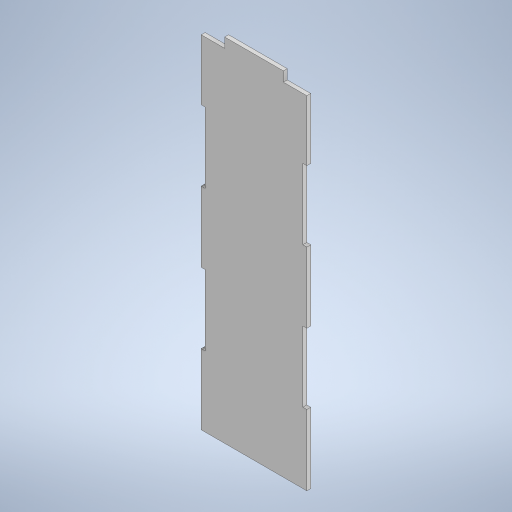
# Autodesk Inventor part: front_side
Saved by Autodesk Inventor 2023 (Build 270158000, 158)
## iProperties
Created: 2023-04-26
Part Number: front_side
Material: Generic
Document SubType Name: Modeling
Designer: Unnar
Density: 1 g/cm^3
Appearance: Default
Author: Unnar
Autodesk Inventor part; units mm, degrees
ref_plane "YZ Plane" through (0, 0, 0) normal (1, 0, 0) x (0, 1, 0)
ref_plane "XZ Plane" through (0, 0, 0) normal (0, 1, 0) x (-1, 0, 0)
ref_plane "XY Plane" through (0, 0, 0) normal (0, 0, 1) x (1, 0, 0)
sketch "Sketch1" plane through (0, 0, 0) normal (0, 0, 1) x (1, 0, 0)
  line L0 (-28.8571, 66) -> (25.1429, 66)
  line L1 (25.1429, 66) -> (25.1429, -114)
  line L2 (25.1429, -114) -> (-28.8571, -114)
  line L3 (-28.8571, -114) -> (-28.8571, 66)
  point P0 (0, 0)
  dimension "d0" = 54
  dimension "d1" = 180
  constraints: 8 end point, 2 parallel, 1 horizontal, 1 perpendicular
  measures "d0" distance of L0.start L0.end
  measures "d1" distance of L0.end L1.end
extrude "Extrusion1" add sketch "Sketch1" along normal blind 2
sketch "Sketch2" plane through (0, 0, 2) normal (0, 0, 1) x (1, 0, 0)
  line L0 (25.1429, 66) -> (-28.8571, 66) projected
  line L1 (-28.8571, 66) -> (-16.8571, 66)
  line L2 (-16.8571, 66) -> (-16.8571, 61)
  line L3 (-16.8571, 61) -> (-28.8571, 61)
  line L4 (-28.8571, 61) -> (-28.8571, 66)
  line L5 (25.1429, 66) -> (13.1429, 66)
  line L6 (13.1429, 66) -> (13.1429, 61)
  line L7 (13.1429, 61) -> (25.1429, 61)
  line L8 (25.1429, 61) -> (25.1429, 66)
  point P0 (0, 0)
  dimension "d4" = 12
  dimension "d5" = 12
  dimension "d6" = 5
  constraints: 16 end point, 4 parallel, 2 horizontal, 2 perpendicular, 1 point on line
  measures "d4" distance of L6.end L7.end
  measures "d5" distance of L2.end L3.end
  measures "d6" distance of L3.end L0.end
extrude "Extrusion2" cut sketch "Sketch2" against normal blind 2
sketch "Sketch3" plane through (0, 0, 2) normal (0, 0, 1) x (1, 0, 0)
  line L0 (-28.8571, 61) -> (-28.8571, -114) projected
  line L1 (-28.8571, 30) -> (-26.8571, 30)
  line L2 (-26.8571, 30) -> (-26.8571, -6)
  line L3 (-26.8571, -6) -> (-28.8571, -6)
  line L4 (-28.8571, -6) -> (-28.8571, 30)
  line L5 (-28.8571, -42) -> (-26.8571, -42)
  line L6 (-26.8571, -42) -> (-26.8571, -78)
  line L7 (-26.8571, -78) -> (-28.8571, -78)
  line L8 (-28.8571, -78) -> (-28.8571, -42)
  line L9 (25.1429, -114) -> (25.1429, 61) projected
  line L10 (25.1429, 30) -> (23.1429, 30)
  line L11 (23.1429, 30) -> (23.1429, -6)
  line L12 (23.1429, -6) -> (25.1429, -6)
  line L13 (25.1429, -6) -> (25.1429, 30)
  line L14 (25.1429, -42) -> (23.1429, -42)
  line L15 (23.1429, -42) -> (23.1429, -78)
  line L16 (23.1429, -78) -> (25.1429, -78)
  line L17 (25.1429, -78) -> (25.1429, -42)
  line L18 (-16.8571, 61) -> (-28.8571, 61) projected
  line L19 (-28.8571, -114) -> (25.1429, -114) projected
  point P0 (0, 0)
  point P1 (-27.8571, 30)
  point P2 (-27.8571, -42)
  point P3 (-27.8571, -6)
  point P4 (-26.8571, -60)
  point P5 (-27.8571, -78)
  dimension "d10" = 36
  dimension "d11" = 36
  dimension "d12" = 2
  dimension "d13" = 2
  dimension "d14" = 36
  dimension "d15" = 36
  constraints: 32 end point, 10 point on line, 8 parallel, 5 midpoint, 4 horizontal, 4 perpendicular
  measures "d10" distance of L1.end L2.end
  measures "d11" distance of point (-27.857, -42) point (-27.857, -6)
  measures "d12" distance from line of L8 point (-26.857, -60)
  measures "d13" distance between parallel lines of L9 L15
  measures "d14" distance of L5.end L6.end
  measures "d15" distance from line of L19 point (-27.857, -78)
extrude "Extrusion3" cut sketch "Sketch3" against normal blind 2
body "Solid1"
